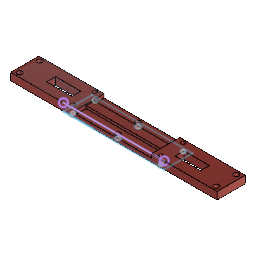
motorhalterung+v17 (Autodesk Fusion 360 design; units mm, degrees)
Autodesk Fusion 360 part; units mm, degrees
note: some values were not read from the file. Chosen so that the rebuilt part matches the saved one: which face or edge a step refers to; that a step has no effect.
sketch "Skizze2" plane through (0, 0, 0) normal (0, 0, 1) x (1, 0, 0)
  circle A0 centre (-10.6288, -6.58) radius 1.5
  circle A1 centre (-10.6288, 10.92) radius 1.5
  line L0 (-15.6288, -9.08) -> (64.3712, -9.08)
  line L1 (64.3712, -9.08) -> (64.3712, 13.42)
  line L2 (64.3712, 13.42) -> (-15.6288, 13.42)
  line L3 (-15.6288, 13.42) -> (-15.6288, -9.08)
  circle A2 centre (59.3712, 10.92) radius 1.5
  circle A3 centre (59.3712, -6.58) radius 1.5
  circle A4 centre (24.3712, 10.17) radius 2
  circle A5 centre (24.3712, -5.83) radius 2
  point P0 (-10.6288, 11.8843)
  dimension "d3" = 3
  dimension "d4" = 3
  dimension "d5" = 17.5
  dimension "d16" = 80
  dimension "d17" = 22.5
  dimension "d22" = 3
  dimension "d24" = 5
  dimension "d25" = 3
  dimension "d26" = 2.5
  dimension "d27" = 5
  dimension "d96" = 4
  dimension "d98" = 3.25
  dimension "d99" = 4
  dimension "d100" = 16
  dimension "d103" = 2.5
  dimension "d118" = 2.5
  dimension "d119" = 2.5
  dimension "d120" = 3.25
  dimension "d121" = 17.5
  dimension "d122" = 5
  dimension "d123" = 5
  constraint horizontal L0
  constraint vertical L1
  constraint horizontal L2
  constraint vertical L3
  measures "d3" diameter of A0
  measures "d4" diameter of A1
  measures "d5" vertical distance of A0.centre A1.centre
  measures "d16" distance of L0.start L0.end
  measures "d17" distance of L0.start L2.end
  measures "d22" diameter of A2
  measures "d24" distance of L1 A2.centre
  measures "d25" diameter of A3
  measures "d26" distance of L0 A3.centre
  measures "d27" distance of L1 A3.centre
  measures "d96" diameter of A4
  measures "d98" distance of L2 A4.centre
  measures "d99" diameter of A5
  measures "d100" distance of A4.centre A5.centre
  measures "d103" distance of A1.centre L2
  measures "d118" distance of L2 A2.centre
  measures "d119" distance of A0.centre L0
  measures "d120" distance of L0 A5.centre
  measures "d121" distance of A2.centre A3.centre
  measures "d122" distance of A0.centre L3
  measures "d123" distance of A1.centre L3
extrude "Extrusion14" add sketch "Skizze2" along normal blind 3
box "Grundkörper Quader2" add length 22.5 width 10 height 2 placed x (0, -1, 0) y (1, 0, 0) z (0, 0, 1) at (-15.6288, 13.42, 3)
box "Grundkörper Quader3" add length 22.5 width 10 height 2 placed x (0, -1, 0) y (1, 0, 0) z (0, 0, 1) at (54.3712, 13.42, 3)
extrude "Extrusion15" cut 4 faces at (59.6212, 10.487, 3) (59.8282, -6.1559, 3) (-10.1839, -6.8714, 3) (-10.5241, 10.4539, 3) along direction (0, 0, 1) blind 9
sketch "Skizze7" plane through (0, 0, 0) normal (0, 0, 1) x (1, 0, 0)
extrude "Extrusion16" add 1 faces at (-6.8824, 4.8051, 5) along direction (0, 0, 1) blind 1
extrude "Extrusion17" add 1 faces at (55.6247, -0.465, 5) along direction (0, 0, 1) blind 1
sketch "Skizze8" plane through (0, 0, 3) normal (0, 0, 1) x (-1, 0, 0)
  circle A0 centre (-24.3712, -10.17) radius 2
  circle A1 centre (-24.3712, 5.83) radius 2
  line L0 (-54.3712, 9.08) -> (-54.3712, -13.42)
  line L1 (-54.3712, -13.42) -> (5.6288, -13.42)
  line L2 (5.6288, -13.42) -> (5.6288, 9.08)
  line L3 (5.6288, 9.08) -> (-54.3712, 9.08)
  line L4 (15.6288, 9.08) -> (-64.3712, 9.08)
  line L5 (-64.3712, -13.42) -> (15.6288, -13.42)
  line L6 (5.6288, -5.42) -> (-54.3712, -5.42)
  line L7 (-54.3712, -5.42) -> (-54.3712, 1.08)
  line L8 (-54.3712, 1.08) -> (5.6288, 1.08)
  line L9 (5.6288, 1.08) -> (5.6288, -5.42)
  dimension "d128" = 60
  dimension "d129" = 22.5
  dimension "d130" = 6.5
  dimension "d131" = 8
  constraint horizontal L6
  constraint vertical L7
  constraint horizontal L8
  constraint vertical L9
  constraint coincident L2 L6.start
  measures "d128" distance of L0 L2
  measures "d129" distance of L4 L5
  measures "d130" distance of L6.start L8.end
  measures "d131" distance of L4 L8
extrude "Extrusion18" add sketch "Skizze8" along normal blind 1 contours L0 L2 L6 L7 L8 L9
extrude "Extrusion19" add 1 faces at (64.3712, 5.92, 4) along direction (1, 0, 0) blind 5
extrude "Extrusion20" add 1 faces at (-15.6288, 5.92, 2) along direction (-1, 0, 0) blind 5
extrude "Extrusion21" add 1 faces at (34.3712, 1.0867, 4) along direction (0, 0, 1) blind 1
extrude "Extrusion22" cut 1 faces at (69.3712, 5.92, 4) along direction (-1, 0, 0) blind 8
extrude "Extrusion23" cut 1 faces at (-20.6288, 5.92, 2) along direction (1, 0, 0) blind 8
extrude "Extrusion24" add 1 faces at (-12.6288, 5.92, 2) along direction (-1, 0, 0) blind 4
extrude "Extrusion25" add 1 faces at (61.3712, 5.92, 4) along direction (1, 0, 0) blind 4
sketch "Skizze9" plane through (65.3712, 0, 0) normal (1, 0, 0) x (0, 1, 0)
  line L0 (-9.08, 0) -> (13.42, 0)
  line L1 (13.42, 0) -> (13.42, 6)
  line L2 (13.42, 6) -> (-9.08, 6)
  line L3 (-9.08, 6) -> (-9.08, 0)
  line L4 (-0.33, 6) -> (4.67, 6)
  line L5 (4.67, 6) -> (4.67, 0)
  line L6 (4.67, 0) -> (-0.33, 0)
  line L7 (-0.33, 0) -> (-0.33, 6)
  dimension "d148" = 22.5
  dimension "d149" = 5
  dimension "d150" = 8.75
  dimension "d151" = 8.75
  constraint horizontal L4
  constraint vertical L5
  constraint horizontal L6
  constraint vertical L7
  constraint coincident L2 L4.start
  measures "d148" distance of L1.end L2.end
  measures "d149" distance of L4.start L4.end
  measures "d150" distance of L3 L7
  measures "d151" distance of L1 L5
sketch "Skizze10" plane through (-16.6288, 0, 0) normal (-1, 0, 0) x (0, -1, 0)
  line L0 (-13.42, 0) -> (9.08, 0)
  line L1 (9.08, 0) -> (9.08, 6)
  line L2 (9.08, 6) -> (-13.42, 6)
  line L3 (-13.42, 6) -> (-13.42, 0)
  line L4 (-4.67, 6) -> (0.33, 6)
  line L5 (0.33, 6) -> (0.33, 0)
  line L6 (0.33, 0) -> (-4.67, 0)
  line L7 (-4.67, 0) -> (-4.67, 6)
  dimension "d156" = 5
  dimension "d157" = 8.75
  constraint horizontal L4
  constraint vertical L5
  constraint horizontal L6
  constraint vertical L7
  constraint coincident L2 L4.start
  measures "d156" distance of L4.start L4.end
  measures "d157" distance of L3 L7
extrude "Extrusion26" add sketch "Skizze10" along normal blind 20 contours L0 L2 L3 L7 | L0 L1 L2 L5
extrude "Extrusion27" add sketch "Skizze9" along normal blind 20 contours L0 L2 L3 L7 | L0 L1 L2 L5
box "Grundkörper Quader4" add length 6 width 22.58 height 15 placed x (0, 0, -1) y (0, 1, 0) z (1, 0, 0) at (85.3712, -9.08, 6)
box "Grundkörper Quader5" add length 6 width 22.42 height 15 placed x (0, 0, -1) y (0, -1, 0) z (-1, 0, 0) at (-36.6288, 13.42, 6)
extrude "Extrusion28" add 1 faces at (100.3712, -1.5533, 2) along direction (1, 0, 0) blind 3
extrude "Extrusion29" add 1 faces at (-51.6288, -1.5267, 4) along direction (-1, 0, 0) blind 3
sketch "Skizze13" plane through (0, 0, 6) normal (0, 0, 1) x (-1, 0, 0)
  line L0 (36.6288, 9) -> (36.6288, 9.08)
  line L1 (36.6288, 9.08) -> (5.6288, 9.08)
  line L2 (5.6288, 9.08) -> (5.6288, -13.42)
  line L3 (5.6288, -13.42) -> (54.6288, -13.42)
  line L4 (54.6288, -13.42) -> (54.6288, 9)
  line L5 (54.6288, 9) -> (36.6288, 9)
  line L6 (36.6288, 0.33) -> (36.6288, -4.67)
  line L7 (36.6288, -4.67) -> (16.6288, -4.67)
  line L8 (16.6288, -4.67) -> (16.6288, 0.33)
  line L9 (16.6288, 0.33) -> (36.6288, 0.33)
  circle A0 centre (10.6288, -10.92) radius 1.5
  circle A1 centre (10.6288, 6.58) radius 1.5
sketch "Skizze14" plane through (0, 0, 6) normal (0, 0, 1) x (-1, 0, 0)
  line L0 (15.6288, 9.08) -> (-64.3712, 9.08)
sketch "Skizze15" plane through (0, 0, 0) normal (0, 0, -1) x (1, 0, 0)
  line L0 (-36.6288, 0.33) -> (-16.6288, 0.33)
  line L1 (-16.6288, 0.33) -> (-16.6288, -4.67)
  line L2 (-16.6288, -4.67) -> (-36.6288, -4.67)
  line L3 (-36.6288, -4.67) -> (-36.6288, 0.33)
  line L4 (85.3712, -4.67) -> (65.3712, -4.67)
  line L5 (65.3712, -4.67) -> (65.3712, 0.33)
  line L6 (65.3712, 0.33) -> (85.3712, 0.33)
  line L7 (85.3712, 0.33) -> (85.3712, -4.67)
  line L8 (-36.6288, 9) -> (-54.6288, 9)
  line L9 (-54.6288, 9) -> (-54.6288, -13.42)
  line L10 (-54.6288, -13.42) -> (85.3712, -13.42)
  line L11 (85.3712, -13.42) -> (85.3712, -13.5)
  line L12 (85.3712, -13.5) -> (103.3712, -13.5)
  line L13 (103.3712, -13.5) -> (103.3712, 9.08)
  line L14 (103.3712, 9.08) -> (-36.6288, 9.08)
  line L15 (-36.6288, 9.08) -> (-36.6288, 9)
  circle A0 centre (59.3712, 6.58) radius 1.5
  circle A1 centre (-10.6288, -10.92) radius 1.5
  circle A2 centre (59.3712, -10.92) radius 1.5
  circle A3 centre (-10.6288, 6.58) radius 1.5
  circle A4 centre (24.3712, -10.17) radius 2
  circle A5 centre (24.3712, 5.83) radius 2
  circle A6 centre (59.3712, -10.92) radius 1.5
  line L16 (24.3712, 5.83) -> (-53.6288, 5.83)
  line L17 (-53.6288, 5.83) -> (-53.6288, -10.17)
  line L18 (-53.6288, -10.17) -> (24.3712, -10.17)
  line L19 (24.3712, -10.17) -> (24.3712, 5.83)
  circle A7 centre (-53.6288, 5.83) radius 2
  circle A8 centre (-53.6288, -10.17) radius 2
  line L20 (24.3712, 5.83) -> (102.3712, 5.83)
  line L21 (102.3712, 5.83) -> (102.3712, -10.17)
  line L22 (102.3712, -10.17) -> (24.3712, -10.17)
  line L23 (24.3712, -10.17) -> (24.3712, 5.83)
  circle A9 centre (102.3712, 5.83) radius 2
  circle A10 centre (102.3712, -10.17) radius 2
  point P0 (59.3712, 6.58)
  point P1 (59.3712, -10.92)
  point P2 (24.3712, -10.17)
  dimension "d201" = 78
  dimension "d202" = 17
  dimension "d203" = 4
  dimension "d204" = 4
  dimension "d205" = 4
  dimension "d206" = 4
  constraint horizontal L16
  constraint vertical L17
  constraint horizontal L18
  constraint vertical L19
  constraint coincident A5.centre L16.start
  constraint coincident L16.end L17.start
  constraint coincident L17.end L18.start
  constraint horizontal L20
  constraint vertical L21
  constraint horizontal L22
  constraint vertical L23
  constraint coincident L20.end L21.start
  constraint coincident L21.end L22.start
  measures "d201" distance of A5.centre L16.end
  measures "d202" distance of L3 L17
  measures "d203" diameter of A7
  measures "d204" diameter of A8
  measures "d205" diameter of A9
  measures "d206" diameter of A10
extrude "Extrusion31" cut 1 faces at (91.3712, 13.5, 4) along direction (0, -1, 0) up to surface (0.08 mm away)
extrude "Extrusion30" [no effect]
extrude "Extrusion32" add 1 faces at (-54.6288, -1.5267, 4) along direction (-1, 0, 0) blind 2
extrude "Extrusion33" add 1 faces at (103.3712, 5.92, 4) along direction (1, 0, 0) blind 2
extrude "Extrusion34" cut sketch "Skizze15" against normal blind 40 contours L9 L16 L17 A7 | L9 A7 | L16 L17 A7 | L13 A9 | L13 L20 L21 A9 | L9 L17 L18 A8 | L9 A8 | L20 L21 A9 | L17 L18 A8 | L13 A10 | L13 L21 L22 A10 | L21 L22 A10
extrude "Extrusion35" add 1 faces at (105.3712, 5.92, 4) along direction (1, 0, 0) blind 1
extrude "Extrusion36" add 1 faces at (-56.6288, -1.5267, 4) along direction (-1, 0, 0) blind 1
extrude "Extrusion37" add 1 faces at (-50.6288, -9, 4) along direction (0, -1, 0) up to surface (0.08 mm away)
extrude "Extrusion38" cut 2 faces at (-29.9622, -0.33, 4) (78.7045, -0.33, 2) along direction (0, -1, 0) blind 1
extrude "Extrusion39" cut 2 faces at (-29.9622, 4.67, 2) (78.7045, 4.67, 4) along direction (0, 1, 0) blind 1
